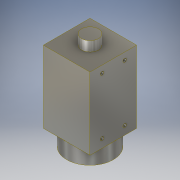
# Autodesk Inventor part: laser
Saved by Autodesk Inventor 2019 (Build 230136000, 136)
## iProperties
Created: 2018-07-12
Part Number: laser
Material: Generic
Document SubType Name: Modeling
Designer: cruiser
Density: 1 g/cm^3
Appearance: Default
Author: cruiser
Autodesk Inventor part; units mm, degrees
ref_plane "YZ Plane" through (0, 0, 0) normal (1, 0, 0) x (0, 1, 0)
ref_plane "XZ Plane" through (0, 0, 0) normal (0, 1, 0) x (-1, 0, 0)
ref_plane "XY Plane" through (0, 0, 0) normal (0, 0, 1) x (1, 0, 0)
sketch "Sketch1" plane through (0, 0, 0) normal (0, 1, 0) x (-1, 0, 0)
  line L0 (-16.5, 16.5) -> (16.5, 16.5)
  line L1 (16.5, 16.5) -> (16.5, -16.5)
  line L2 (16.5, -16.5) -> (-16.5, -16.5)
  line L3 (-16.5, -16.5) -> (-16.5, 16.5)
  line L4 (-16.5, 16.5) -> (16.5, -16.5) construction
  line L5 (16.5, 16.5) -> (-16.5, -16.5) construction
  point P0 (0, 0)
  dimension "d0" = 33
  dimension "d1" = 33
  constraints: 12 end point, 2 midpoint, 2 parallel, 1 horizontal, 1 perpendicular
  measures "d0" distance of L1.end L2.end
  measures "d1" distance of L0.end L1.end
extrude "Extrusion1" add sketch "Sketch1" along normal blind 62
sketch "Sketch2" plane through (0, 62, 0) normal (0, 1, 0) x (1, 0, 0)
  circle A0 centre (0, 0) radius 6
  dimension "d4" = 12
  constraints: 1 centre point, 1 coincident
  measures "d4" diameter of A0
extrude "Extrusion2" add sketch "Sketch2" along normal blind 7
sketch "Sketch3" plane through (16.5, 0, 16.5) normal (1, 0, 0) x (0, 0, -1)
  circle A0 centre (8.5, 57) radius 1.575
  line L0 (-0.0785, 57) -> (33, 57)
  line L1 (33, 0) -> (33, 62) projected
  line L2 (0, 62) -> (33, 62) projected
  line L3 (33, 62) -> (0, 62) projected
  line L4 (16.5, 62) -> (16.5, 57)
  line L5 (0, 17) -> (33, 17)
  line L6 (16.5, 57) -> (16.5, 17)
  line L7 (16.5, 37) -> (33, 37)
  circle A1 centre (24.5, 57) radius 1.575
  circle A2 centre (8.5, 17) radius 1.575
  circle A3 centre (24.5, 17) radius 1.575
  point P0 (16.5, 0)
  dimension "d7" = 3.15
  dimension "d8" = 5
  dimension "d9" = 8
  dimension "d10" = 40
  constraints: 10 end point, 5 point on line, 4 centre point, 3 midpoint, 3 symmetric about line, 2 horizontal, 2 perpendicular, 3 other
  measures "d7" diameter of A0
  measures "d8" distance between parallel lines of L2 L0
  measures "d9" distance from line of L4 A0.centre
  measures "d10" distance between parallel lines of L0 L5
hole "Hole1" at (16.5, 57, 8) at (16.5, 57, -8) at (16.5, 17, 8) at (16.5, 17, -8) direction (-1, 0, 0) diameter 2.459 depth 10 tip angle 118 thread size "M3x0.5" class "6H" standard "ANSI Metric M Profile"
sketch "Sketch4" plane through (0, 0, 0) normal (0, -1, 0) x (1, 0, 0)
  circle A0 centre (0, 0) radius 16.5
  line L0 (16.5, -16.5) -> (-16.5, -16.5) projected
  line L1 (-16.5, 16.5) -> (16.5, 16.5)
  line L2 (16.5, 16.5) -> (16.5, -16.5)
  line L3 (16.5, -16.5) -> (-16.5, -16.5)
  line L4 (-16.5, -16.5) -> (-16.5, 16.5)
  line L5 (-16.5, 16.5) -> (16.5, -16.5) construction
  line L6 (16.5, 16.5) -> (-16.5, -16.5) construction
  dimension "d18" = 33
  constraints: 12 end point, 2 midpoint, 2 parallel, 1 centre point, 1 coincident, 1 horizontal, 1 perpendicular
  measures "d18" diameter of A0
extrude "Extrusion3" cut sketch "Sketch4" against normal blind 11 contours L2 L0 A0 | A0 L1 L2 | A0 L4 L1 | L0 L4 A0
equation "\"d0\" = laser_y"
equation "\"d1\" = laser_z"
equation "\"d2\" = laser_x"
equation "\"d4\" = laser_diameter"
equation "\"d7\" = m3_diameter"
equation "\"d10\" = laser_screw_spacing_x"
equation "\"d18\" = laser_y"
equation "\"thick_acrylic\" = 5.88"
equation "\"thin_acrylic\" = 3.15"
equation "\"clear_acrylic\" = 3.15"
equation "\"wood_thickness\" = 6.72"
equation "\"al1_thickness\" = 1.5875"
equation "\"m3_diameter\" = 3.15"
equation "\"m4_diameter\" = 4.2"
equation "\"m5_diameter\" = 5.25"
equation "\"brass_insert_drill\" = 4"
equation "\"m5_brass_insert_drill\" = 6.7"
equation "\"m5_press_nut_drill\" = 6.35"
equation "\"m3_main_length\" = 14"
equation "\"m3_main_nut_width\" = 5.7"
equation "\"m3_main_nut_thickness\" = 2.5"
equation "\"m3_main_extra\" = 1"
equation "\"stepper_screw_space\" = 35"
equation "\"stepper_shaft_diameter\" = 5"
equation "\"stepper_body_diameter\" = 28"
equation "\"laser_body_diameter\" = 12"
equation "\"t_carrier\" = 6.72"
equation "\"t_wall\" = 5.88"
equation "\"t_window\" = 3.15"
equation "\"carrier_y\" = 181"
equation "\"carrier_z\" = 233.04"
equation "\"carrier_z2\" = 283.04"
equation "\"protection_slot\" = 30.2"
equation "\"protection_slot_offset\" = 37.75"
equation "\"protection_slot_length\" = 20.6"
equation "\"window_z\" = 185"
equation "\"window_y\" = 49.56"
equation "\"window_slot\" = 25"
equation "\"door_sensor\" = 35"
equation "\"reservoir_x\" = 151"
equation "\"reservoir_y\" = 151"
equation "\"linear_bearing_spacing\" = 207"
equation "\"linear_bearing_z\" = 304.8"
equation "\"threaded_rod_z\" = 203.2"
equation "\"motor_spacing\" = 287"
equation "\"t_tray\" = 3.15"
equation "\"tray_border\" = 15"
equation "\"tray_x\" = 151"
equation "\"tray_y\" = 181"
equation "\"bed_t\" = 1.5875"
equation "\"bed_y2\" = 45.96"
equation "\"bed_fold_x\" = 15"
equation "\"bed_gap\" = 0.3"
equation "\"t_inner_tray\" = 5.88"
equation "\"t_tape\" = 3"
equation "\"inner_tray_x\" = 145"
equation "\"inner_tray_y\" = 145"
equation "\"inner_tray_border\" = 5"
equation "\"inner_tray_radius\" = 24"
equation "\"t_bottom_clear\" = 3.15"
equation "\"bottom_clear_border\" = 5"
equation "\"brass_keep_out\" = 8"
equation "\"tape_keep_out\" = 2"
equation "\"tape_thickness\" = 2"
equation "\"t_crane\" = 6.72"
equation "\"crane_x\" = 244.56"
equation "\"end_stop_offset_x\" = 83"
equation "\"end_stop_spacing\" = 19"
equation "\"thumb_nut_offset_y\" = 11.72"
equation "\"thumb_nut_diameter\" = 7"
equation "\"z_min_from_center\" = 72.28"
equation "\"t_frame\" = 6.72"
equation "\"frame_top_z\" = 295"
equation "\"frame_bottom_z\" = 225"
equation "\"frame_y\" = 68.44"
equation "\"frame_border\" = 39.5"
equation "\"frame_foot_z\" = 49.5"
equation "\"frame_foot_extension\" = 6"
equation "\"frame_tilt\" = 0"
equation "\"printer_z\" = 289"
equation "\"lcd_x\" = 72"
equation "\"lcd_y\" = 25"
equation "\"subframe_y_offset\" = 27.5"
equation "\"laser_y_offset\" = 19.4"
equation "\"laser_diameter\" = 12"
equation "\"laser_y\" = 33"
equation "\"laser_z\" = 33"
equation "\"laser_x\" = 62"
equation "\"laser_screw_spacing_x\" = 40"
equation "\"laser_screw_spacing_y\" = 16"
equation "\"t_galvo_frame\" = 6.72"
equation "\"galvo_frame_x\" = 66"
equation "\"galvo_frame_z\" = 65"
equation "\"galvo_frame_y_offset\" = 27.5"
equation "\"drawer_x\" = 181"
equation "\"drawer_y\" = 49.56"
equation "\"drawer_z\" = 206.72"
equation "\"drawer_z_from_bottom\" = 25"
equation "\"drawer_foot_mount\" = 18"
equation "\"asym_key\" = 0"
equation "\"small_round\" = 2"
body "Solid1"
